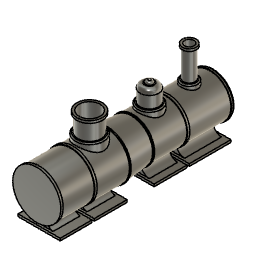
Steam Engine (Autodesk Fusion 360 design; units mm, degrees)
Autodesk Fusion 360 part; units mm, degrees
sketch "Sketch1" plane through (0, 0, 0) normal (0, 1, 0) x (1, 0, 0) in component "Component"
  circle A0 centre (0, 0) radius 20
  circle A1 centre (0, 0) radius 18
  circle A2 centre (0, 0) radius 20.5
  circle A3 centre (0, 0) radius 18.5
  line L0 (6.5, 0) -> (3.25, 5.6292)
  line L1 (3.25, 5.6292) -> (-3.25, 5.6292)
  line L2 (-3.25, 5.6292) -> (-6.5, 0)
  line L3 (-6.5, 0) -> (-3.25, -5.6292)
  line L4 (-3.25, -5.6292) -> (3.25, -5.6292)
  line L5 (3.25, -5.6292) -> (6.5, 0)
  dimension "d1" = 40
  dimension "d2" = 36
  dimension "d3" = 41
  dimension "d4" = 37
  dimension "d5" = 6.5
  constraint coincident A0.centre A1.centre
  constraint concentric A0 A2
  constraint concentric A1 A3
  measures "d1" diameter of A0
  measures "d2" diameter of A1
  measures "d3" diameter of A2
  measures "d4" diameter of A3
  measures "d5" distance of L0.start A0.centre
extrude "Extrude12" add sketch "Sketch1" against normal blind 60 contours A0 | A1 | A3 | L0 L1 L2 L3 L4 L5 in component "Component"
extrude "Extrude13" add sketch "Sketch1" along normal blind 90 contours A1 | L0 L1 L2 L3 L4 L5 in component "Component"
extrude "Extrude15" add sketch "Sketch1" against normal blind 60 contours A2 in component "Component"
extrude "Extrude16" cut sketch "Sketch1" against normal blind 58 contours A2 in component "Component"
extrude "Extrude17" add sketch "Sketch1" against normal blind 31 contours A2 in component "Component"
extrude "Extrude18" cut sketch "Sketch1" against normal blind 29 contours A2 in component "Component"
extrude "Extrude19" add sketch "Sketch1" against normal blind 1 contours A2 in component "Component"
extrude "Extrude20" add sketch "Sketch1" along normal blind 92.5 contours L0 L1 L2 L3 L4 L5 in component "Component"
extrude "Extrude21" add sketch "Sketch1" along normal blind 89 contours A3 in component "Component"
extrude "Extrude22" cut sketch "Sketch1" along normal blind 87.5 contours A3 in component "Component"
extrude "Extrude23" add sketch "Sketch1" along normal blind 52 contours A3 in component "Component"
extrude "Extrude24" cut sketch "Sketch1" along normal blind 50 contours A3 in component "Component"
extrude "Extrude26" cut sketch "Sketch1" along normal blind 16 contours A3 in component "Component"
extrude "Extrude27" add sketch "Sketch1" along normal blind 22 contours A3 in component "Component"
extrude "Extrude28" cut sketch "Sketch1" along normal blind 21 contours A3 in component "Component"
extrude "Extrude29" add sketch "Sketch1" along normal blind 36 draft -5.5 contours A0 | A1 | A3 | L0 L1 L2 L3 L4 L5 in component "Component"
sketch "Sketch2" plane through (0, 0, 0) normal (0, 0, 1) x (1, 0, 0) in component "Component"
  circle A0 centre (0, 70) radius 7
  circle A1 centre (0, 70) radius 6
  circle A2 centre (0, 70) radius 5
  circle A3 centre (0, -15) radius 12
  circle A4 centre (0, -15) radius 11
  circle A5 centre (0, -15) radius 10
  circle A6 centre (0, 36) radius 10
  circle A7 centre (0, 36) radius 9
  circle A8 centre (0, 36) radius 8
  circle A9 centre (0, 36) radius 3
  dimension "d65" = 70
  dimension "d66" = 14
  dimension "d67" = 12
  dimension "d68" = 10
  dimension "d87" = 24
  dimension "d88" = 15
  dimension "d89" = 22
  dimension "d90" = 20
  dimension "d107" = 20
  dimension "d108" = 36
  dimension "d109" = 18
  dimension "d110" = 16
  dimension "d124" = 6
  constraint concentric A0 A1
  constraint concentric A0 A2
  constraint concentric A3 A4
  constraint concentric A4 A5
  constraint concentric A6 A7
  constraint concentric A7 A8
  constraint concentric A7 A9
  measures "d65" distance of origin A0.centre
  measures "d66" diameter of A0
  measures "d67" diameter of A1
  measures "d68" diameter of A2
  measures "d87" diameter of A3
  measures "d88" distance of origin A3.centre
  measures "d89" diameter of A4
  measures "d90" diameter of A5
  measures "d107" diameter of A6
  measures "d108" distance of origin A6.centre
  measures "d109" diameter of A7
  measures "d110" diameter of A8
  measures "d124" diameter of A9
extrude "Extrude41" cut sketch "Sketch2" along normal blind 25 contours A6 | A7 | A8 | A9 in component "Component"
extrude "Extrude30" cut sketch "Sketch2" along normal blind 25 contours A0 | A1 | A2 in component "Component"
extrude "Extrude31" add sketch "Sketch2" along normal blind 47 contours A2 in component "Component"
extrude "Extrude33" add sketch "Sketch2" along normal blind 20 contours A0 in component "Component"
extrude "Extrude34" add sketch "Sketch2" along normal blind 21 contours A1 in component "Component"
fillet "Fillet1" radius 1 1 edges at (-5.594, 72.1697, 20) in component "Component"
hole "Hole1" at (0, 70, 47) direction (0, 0, -1) diameter 8 depth 26 tip angle 180 in component "Component"
sketch "Sketch3" plane through (0, 0, 47) normal (0, 0, 1) x (-1, 0, 0) in component "Component"
  circle A0 centre (0, -70) radius 4
  circle A1 centre (0, -70) radius 5
  circle A2 centre (0, -70) radius 6
  circle A3 centre (0, -70) radius 5
  dimension "d83" = 12
  dimension "d84" = 10
  constraint concentric A0 A2
  constraint concentric A2 A3
  measures "d83" diameter of A2
  measures "d84" diameter of A3
extrude "Extrude35" add sketch "Sketch3" against normal blind 2 contours A2 in component "Component"
extrude "Extrude36" cut sketch "Sketch2" along normal blind 30 contours A3 | A4 | A5 in component "Component"
extrude "Extrude37" add sketch "Sketch2" along normal blind 23 contours A3 in component "Component"
extrude "Extrude38" add sketch "Sketch2" along normal blind 24 contours A4 in component "Component"
fillet "Fillet2" radius 1 1 edges at (-10.2556, -11.0222, 23) in component "Component"
extrude "Extrude39" add sketch "Sketch2" along normal blind 40 contours A5 in component "Component"
hole "Hole2" at (0, -15, 40) direction (0, 0, -1) diameter 18 depth 16 tip angle 180 in component "Component"
sketch "Sketch4" plane through (0, 0, 40) normal (0, 0, 1) x (-1, 0, 0) in component "Component"
  circle A0 centre (0, 15) radius 9
  circle A1 centre (0, 15) radius 10
  circle A2 centre (0, 15) radius 10
  circle A3 centre (0, 15) radius 11
  dimension "d103" = 20
  dimension "d104" = 22
  constraint concentric A0 A2
  constraint concentric A2 A3
  measures "d103" diameter of A2
  measures "d104" diameter of A3
extrude "Extrude40" add sketch "Sketch4" against normal blind 2 contours A3 in component "Component"
extrude "Extrude42" add sketch "Sketch2" along normal blind 20 contours A6 in component "Component"
extrude "Extrude43" add sketch "Sketch2" along normal blind 21 contours A7 in component "Component"
extrude "Extrude44" add sketch "Sketch2" along normal blind 35 contours A8 | A9 in component "Component"
fillet "Fillet3" radius 1 1 edges at (-8.3909, 39.2545, 20) in component "Component"
fillet "Fillet4" radius 4 1 edges at (-7.4586, 33.1071, 35) in component "Component"
extrude "Extrude45" add sketch "Sketch2" along normal blind 37 contours A9 in component "Component"
fillet "Fillet5" radius 2 1 edges at (-2.797, 34.9152, 37) in component "Component"
sphere "SpherePrimitive1" add diameter 2 placed x (-1, 0, 0) y (0, -1, 0) z (0, 0, 1) at (0, 36, 37) in component "Component"
sketch "Sketch8" plane through (0, 90, 0) normal (0, 1, 0) x (-1, 0, 0) in component "Component"
  line L0 (-3.25, 5.6292) -> (3.25, 5.6292)
  line L1 (3.25, 5.6292) -> (6.5, 0)
  line L2 (6.5, 0) -> (3.25, -5.6292)
  line L3 (3.25, -5.6292) -> (-3.25, -5.6292)
  line L4 (-3.25, -5.6292) -> (-6.5, 0)
  line L5 (-6.5, 0) -> (-3.25, 5.6292)
  circle A0 centre (0, 0) radius 18
  circle A1 centre (0, 0) radius 18
  line L6 (0, -26) -> (18, -26)
  line L7 (18, -26) -> (-18, -26)
  line L8 (-18, -26) -> (-18, -24)
  line L9 (-18, -24) -> (18, -24)
  line L10 (18, -24) -> (18, -26)
  line L11 (0, -24) -> (5, -24)
  line L12 (5, -24) -> (5, -17.2916)
  line L13 (0, -24) -> (-5, -24)
  line L14 (-5, -24) -> (-5, -17.2916)
  circle A2 centre (0, 0) radius 18.5
  circle A3 centre (0, 0) radius 8.75
  circle A4 centre (0, 0) radius 16
  circle A5 centre (0, 0) radius 15
  line L15 (6.5, 0) -> (3.25, 5.6292)
  line L16 (3.25, 5.6292) -> (-3.25, 5.6292)
  line L17 (-3.25, 5.6292) -> (-6.5, 0)
  line L18 (-6.5, 0) -> (-3.25, -5.6292)
  line L19 (-3.25, -5.6292) -> (3.25, -5.6292)
  line L20 (3.25, -5.6292) -> (6.5, 0)
  dimension "d161" = 36
  dimension "d162" = 26
  dimension "d163" = 18
  dimension "d164" = 36
  dimension "d165" = 2
  dimension "d166" = 5
  dimension "d168" = 5
  dimension "d174" = 37
  dimension "d228" = 17.5
  dimension "d229" = 32
  dimension "d230" = 30
  dimension "d231" = 6.5
  constraint coincident A0.centre A1.centre
  constraint horizontal L6
  constraint horizontal L7
  constraint vertical L8
  constraint horizontal L9
  constraint vertical L10
  constraint horizontal L11
  constraint midpoint L9 L11.start
  constraint vertical L12
  constraint horizontal L13
  constraint vertical L14
  constraint coincident A0 L14.end
  constraint coincident A0 L12.end
  constraint concentric A1 A3
  constraint concentric A3 A4
  constraint concentric A4 A5
  measures "d161" diameter of A1
  measures "d162" distance of A0.centre L6.start
  measures "d163" distance of L6.start L6.end
  measures "d164" distance of L6.end L7.end
  measures "d165" distance of L6.end L9.end
  measures "d166" distance of L11.start L11.end
  measures "d168" distance of L11.start L13.end
  measures "d174" diameter of A2
  measures "d228" diameter of A3
  measures "d229" diameter of A4
  measures "d230" diameter of A5
  measures "d231" distance of L1.end A0.centre
extrude "Extrude55" add sketch "Sketch8" against normal blind 66 contours A0 A1 L12 L14 A2 | L9 L11 L12 L13 L14 A2 picked at (-4.175, -17.6417) in component "Component"
extrude "Extrude56" cut sketch "Sketch8" against normal blind 42 contours A0 A1 L12 L14 A2 | L9 L11 L12 L13 L14 A2 picked at (-4.175, -17.6417) in component "Component"
extrude "Extrude57" add sketch "Sketch8" against normal blind 40 contours A0 A1 L12 L14 A2 picked at (-4.175, -17.6417) in component "Component"
extrude "Extrude58" cut sketch "Sketch8" against normal blind 38 contours A0 A1 L12 L14 A2 picked at (-4.175, -17.6417) in component "Component"
extrude "Extrude59" add sketch "Sketch8" against normal blind 36 contours A0 A1 L12 L14 A2 | L9 L11 L12 L13 L14 A2 picked at (-4.175, -17.6417) in component "Component"
extrude "Extrude60" cut sketch "Sketch8" against normal blind 4.5 contours A0 A1 L12 L14 A2 | L9 L11 L12 L13 L14 A2 picked at (-4.175, -17.6417) in component "Component"
extrude "Extrude61" add sketch "Sketch8" against normal blind 2.5 contours A0 A1 L12 L14 A2 picked at (-4.175, -17.6417) in component "Component"
extrude "Extrude62" cut sketch "Sketch8" against normal blind 1 contours A0 A1 L12 L14 A2 picked at (-4.175, -17.6417) in component "Component"
extrude "Extrude63" add sketch "Sketch8" against normal blind 68 contours L6 L7 L8 L9 L10 L11 L13 in component "Component"
extrude "Extrude64" cut sketch "Sketch8" against normal blind 40 contours L6 L7 L8 L9 L10 L11 L13 in component "Component"
extrude "Extrude65" add sketch "Sketch8" against normal blind 38 contours L6 L7 L8 L9 L10 L11 L13 in component "Component"
extrude "Extrude66" cut sketch "Sketch8" against normal blind 2.5 contours L6 L7 L8 L9 L10 L11 L13 in component "Component"
sketch "Sketch9" plane through (0, -60, 0) normal (0, -1, 0) x (1, 0, 0) in component "Component"
  circle A0 centre (0, 0) radius 20.5
  circle A1 centre (0, 0) radius 20.5
  circle A2 centre (0, 0) radius 20
  line L0 (0, -26) -> (18, -26)
  line L1 (18, -26) -> (-18, -26)
  line L2 (-18, -26) -> (-18, -24)
  line L3 (-18, -24) -> (18, -24)
  line L4 (18, -24) -> (18, -26)
  line L5 (0, -24) -> (5, -24)
  line L6 (5, -24) -> (5, -19.3649)
  line L7 (0, -24) -> (-5, -24)
  line L8 (-5, -24) -> (-5, -19.3649)
  dimension "d195" = 41
  dimension "d196" = 40
  dimension "d197" = 26
  dimension "d198" = 18
  dimension "d199" = 36
  dimension "d200" = 2
  dimension "d201" = 5
  dimension "d202" = 5
  constraint concentric A0 A1
  constraint concentric A1 A2
  constraint horizontal L0
  constraint horizontal L1
  constraint vertical L2
  constraint horizontal L3
  constraint vertical L4
  constraint horizontal L5
  constraint midpoint L3 L5.start
  constraint vertical L6
  constraint horizontal L7
  constraint vertical L8
  constraint coincident A2 L8.end
  constraint coincident A2 L6.end
  measures "d195" diameter of A1
  measures "d196" diameter of A2
  measures "d197" distance of A0.centre L0.start
  measures "d198" distance of L0.start L0.end
  measures "d199" distance of L0.end L1.end
  measures "d200" distance of L0.end L3.end
  measures "d201" distance of L5.start L5.end
  measures "d202" distance of L5.start L7.end
extrude "Extrude67" add sketch "Sketch9" against normal blind 57 contours A0 A1 A2 L6 L8 | A0 A1 L3 L5 L6 L7 L8 picked at (4.1734, -19.6955) in component "Component"
extrude "Extrude68" cut sketch "Sketch9" against normal blind 33 contours A0 A1 A2 L6 L8 | A0 A1 L3 L5 L6 L7 L8 picked at (4.1734, -19.6955) in component "Component"
extrude "Extrude69" add sketch "Sketch9" against normal blind 31 contours A0 A1 A2 L6 L8 picked at (4.1734, -19.6955) in component "Component"
extrude "Extrude70" cut sketch "Sketch9" against normal blind 29 contours A0 A1 A2 L6 L8 picked at (4.1734, -19.6955) in component "Component"
extrude "Extrude71" add sketch "Sketch9" against normal blind 27 contours A0 A1 A2 L6 L8 | A0 A1 L3 L5 L6 L7 L8 picked at (4.1734, -19.6955) in component "Component"
extrude "Extrude72" cut sketch "Sketch9" against normal blind 4 contours A0 A1 A2 L6 L8 | A0 A1 L3 L5 L6 L7 L8 picked at (4.1734, -19.6955) in component "Component"
extrude "Extrude73" add sketch "Sketch9" against normal blind 2 contours A0 A1 A2 L6 L8 picked at (4.1734, -19.6955) in component "Component"
extrude "Extrude74" add sketch "Sketch9" against normal blind 59 contours L0 L1 L2 L3 L4 L5 L7 in component "Component"
extrude "Extrude75" cut sketch "Sketch9" against normal blind 31 contours L0 L1 L2 L3 L4 L5 L7 in component "Component"
extrude "Extrude76" add sketch "Sketch9" against normal blind 29 contours L0 L1 L2 L3 L4 L5 L7 in component "Component"
extrude "Extrude77" cut sketch "Sketch9" against normal blind 2 contours L0 L1 L2 L3 L4 L5 L7 in component "Component"
extrude "Extrude78" cut 1 faces at (-1.0833, 92.5, 1.8764) along direction (0, -1, 0) blind 2.5 in component "Component"
extrude "Extrude79" add sketch "Sketch8" along normal blind 1 contours A4 in component "Component"
extrude "Extrude80" add sketch "Sketch8" along normal blind 2.5 contours L0 L1 L2 L3 L4 L5 L15 L16 L17 L18 L19 L20 | A3 in component "Component"
extrude "Extrude81" add sketch "Sketch8" along normal blind 4.5 contours L0 L1 L2 L3 L4 L5 L15 L16 L17 L18 L19 L20 in component "Component"
sketch "Sketch1 (2)" plane through (0, 0, 0) normal (0, 0, 1) x (1, 0, 0)
  line L0 (4.5, 94.5) -> (11.3595, 93.1044)
  line L1 (4.5, 94.5) -> (11.5, 94.5) construction
  line L2 (11.3595, 93.1044) -> (11.5, 94.5)
  line L3 (11.5, 94.5) -> (4.5, 94.5)
  dimension "d238" = 7
  dimension "d239" = 11.5
  constraint horizontal L1
  constraint parallel L1 L3
  measures "d238" distance of L0.start L0.end
  measures "d239" angle of L0 L1
revolve "Revolve1" cut sketch "Sketch1 (2)" angle 360 about axis through (0, 1.75, 0) along (0, 1, 0) in component "Component"
fillet "Fillet7" radius 7 4 edges at (5, 36, -24) (5, 69.75, -24) (-5, 36, -24) (-5, 69.75, -24) in component "Component"
fillet "Fillet8" radius 5 4 edges at (-5, -15, -24) (-5, -44.5, -24) (5, -44.5, -24) (5, -15, -24) in component "Component"
sketch "Sketch2 (2)" plane through (0, 94.5, 0) normal (0, 1, 0) x (-1, 0, 0)
  circle A0 centre (0, 0) radius 4.5
  line L0 (-3.3729, -1.4406) -> (3.2697, -1.4406) construction
  line L1 (3.2697, -1.4406) -> (3.2697, 2.5594) construction
  line L2 (3.2697, 2.5594) -> (-3.3729, 2.5594) construction
  line L3 (-3.3729, 2.5594) -> (-3.3729, -1.4406) construction
  text T0 "486" font "Arial" height 4 bold italic align ink ink in box 0 x 0 at (-3.3729, -1.4406) x (1, 0) y (0, 1) spacing 1 height is em
  constraint perpendicular L0 L1
  constraint parallel L0 L2
  constraint parallel L1 L3
extrude "Extrude82" add sketch "Sketch2 (2)" along normal blind 1 text T0 in component "Component"
component "Component" placed x (1, 0, 0) y (0, 1, 0) z (0, 0, 1) at (0, 0, 0)
equation "d50 = 37 mm + 15 mm"
equation "d181 = -2.5 mm - 2 mm"
equation "d193 = -4.5 mm + 2 mm"
